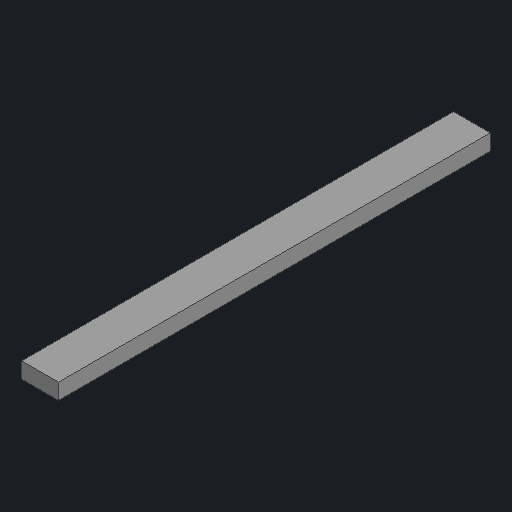
# Autodesk Inventor part: 2x4x42
Saved by Autodesk Inventor 2027.1 (Build 311270010, 270A)
## iProperties
Created: 2024-09-20
Part Number: 2x4x42
Material: Generic
Document SubType Name: Modeling
Designer: User
Density: 1 g/cm^3
Appearance: Default
Finish1_Area: 420.500 in^2
Finish1_Appearance: Red
Finish1_Process: Prime/Paint RAL 3018
Finish1_Description: Prime/Paint RAL 3018
Finish1_ShortDescription: RAL 3018
Finish1_Thickness: 0.002 in
Author: User
Autodesk Inventor part; units mm, degrees
ref_plane "YZ Plane" through (0, 0, 0) normal (1, 0, 0) x (0, 1, 0)
ref_plane "XZ Plane" through (0, 0, 0) normal (0, 1, 0) x (-1, 0, 0)
ref_plane "Work Plane1" through (-322.8193, 0, 0) normal (0, 0, 1) x (1, 0, 0)
sketch "Sketch1" plane through (-322.8193, 0, 0) normal (0, 0, 1) x (1, 0, 0)
  line L0 (322.8193, 0) -> (411.7193, 0)
  line L1 (411.7193, 0) -> (411.7193, -38.1)
  line L2 (411.7193, -38.1) -> (322.8193, -38.1)
  line L3 (322.8193, -38.1) -> (322.8193, 0)
  dimension "d0" = 38.1
  dimension "d1" = 88.9
  constraints: 8 end point, 2 parallel, 1 horizontal, 1 perpendicular
  measures "d0" distance of L0.end L1.end
  measures "d1" distance of L1.end L2.end
extrude "Extrusion1" add sketch "Sketch1" along normal blind 1041.4
body "Solid1"
